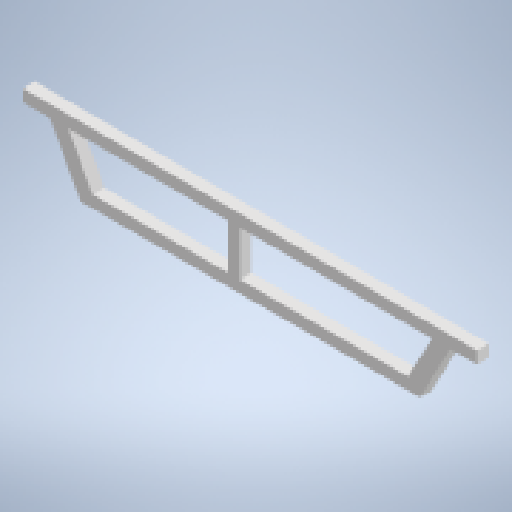
# Autodesk Inventor part: DOF8
Saved by Autodesk Inventor 2024 (Build 280153000, 153)
## iProperties
Created: 2024-10-16
Part Number: DOF8
Material: 一般
Document SubType Name: Modeling
Designer: jerry
Density: 1 g/cm^3
Appearance: 預設
Author: jerry
Autodesk Inventor part; units mm, degrees
ref_plane "YZ Plane" through (0, 0, 0) normal (1, 0, 0) x (0, 1, 0)
ref_plane "XZ Plane" through (0, 0, 0) normal (0, 1, 0) x (-1, 0, 0)
ref_plane "XY Plane" through (0, 0, 0) normal (0, 0, 1) x (1, 0, 0)
sketch "草圖1" plane through (0, 0, 0) normal (0, 0, 1) x (1, 0, 0)
  line L0 (0, 0) -> (0, -20)
  line L1 (0, -20) -> (-115, -20)
  line L2 (0, -20) -> (450, -20)
  line L3 (167.5, 0) -> (430, 0)
  line L4 (167.5, 0) -> (-95, 0)
  line L5 (167.5, 75) -> (470, 75)
  line L6 (470, 75) -> (430, 0)
  line L7 (167.5, 75) -> (-135, 75)
  line L8 (-135, 75) -> (-95, 0)
  line L9 (130, 0) -> (130, 75)
  line L10 (130, 0) -> (150, 0)
  line L11 (150, 0) -> (150, 75)
  line L12 (167.5, 95) -> (545, 95)
  line L13 (545, 95) -> (545, 75)
  line L14 (545, 75) -> (500, 75)
  line L15 (500, 75) -> (450, -20)
  line L16 (-115, -20) -> (-165.6667, 75)
  line L17 (-165.6667, 75) -> (-210.6667, 75)
  line L18 (-210.6667, 75) -> (-210.6667, 95)
  line L19 (-210.6667, 95) -> (167.5, 95)
  dimension "d0" = 20
  dimension "d1" = 115
  dimension "d2" = 450
  dimension "d6" = 262.5
  dimension "d7" = 262.5
  dimension "d8" = 302.5
  dimension "d9" = 302.5
  dimension "d11" = 20
  dimension "d12" = 75
  dimension "d14" = 377.5
  dimension "d15" = 20
  dimension "d16" = 45
  dimension "d17" = 45
  dimension "d18" = 20
  constraints: 40 end point, 7 point on line, 5 horizontal, 5 perpendicular, 1 parallel, 1 vertical
  measures "d0" distance of L0.start L0.end
  measures "d1" distance of L0.end L1.end
  measures "d2" distance of L0.end L2.end
  measures "d6" distance of L3.start L3.end
  measures "d7" distance of L3.start L4.end
  measures "d8" distance of L5.start L5.end
  measures "d9" distance of L5.start L7.end
  measures "d11" distance of L9.start L10.end
  measures "d12" distance of L10.end L11.end
  measures "d14" distance of L12.start L12.end
  measures "d15" distance of L12.end L13.end
  measures "d16" distance of L13.end L14.end
  measures "d17" distance of L16.end L17.end
  measures "d18" distance of L17.end L18.end
extrude "擠出1" add sketch "草圖1" along normal blind 20 contours L1 L16 L17 L18 L19 L12 L13 L14 L15 L2 | L9 L7 L11 L4
sketch "草圖2" plane through (-210.6667, 95, 0) normal (0, 1, 0) x (1, 0, 0)
  line L0 (0, 0) -> (0, -20) projected
  circle A0 centre (0, -10) radius 32.5
  circle A1 centre (32.5, -10) radius 5
  line L1 (755.6667, 0) -> (755.6667, -20) projected
  circle A2 centre (755.6667, -10) radius 32.5
  circle A3 centre (723.1667, -10) radius 5
  point P0 (210.6667, 0)
  dimension "d21" = 65
  dimension "d23" = 65
  dimension "d22" = 10
  dimension "d24" = 10
  constraints: 2 centre point, 2 horizontal alignment, 2 midpoint, 4 other
  measures "d22" diameter of A1
  measures "d24" diameter of A3
extrude "擠出2" add sketch "草圖2" along normal blind 20 contours A0 A1 | A0 A1 | A3 A2 | A2 A3 picked at (30.8705, -10.9665) picked at (33.9711, -11.3119) picked at (724.8619, -10) picked at (721.5286, -10)
sketch "草圖3" plane through (512.5, 115, 10) normal (0, 1, 0) x (1, 0, 0)
  circle A0 centre (0, 0) radius 17.5
  point P0 (-512.5, 10)
  dimension "d27" = 35
  constraints: 1 centre point
  measures "d27" diameter of A0
extrude "擠出3" add sketch "草圖3" along normal blind 10
sketch "草圖4" plane through (-178.1667, 115, 10) normal (0, 1, 0) x (1, 0, 0)
  circle A0 centre (0, 0) radius 5 projected
  circle A1 centre (0, 0) radius 17.5
  point P0 (178.1667, 10)
  dimension "d30" = 35
  constraints: 1 centre point, 1 coincident
  measures "d30" diameter of A1
extrude "擠出4" add sketch "草圖4" along normal blind 10 contours A0 | A1
